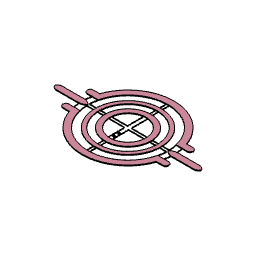
ホシノ_ヘイロー_mk1 v4 (Autodesk Fusion 360 design; units mm, degrees)
Autodesk Fusion 360 part; units mm, degrees
sketch "スケッチ1" plane through (0, 0, 0) normal (0, 0, 1) x (1, 0, 0)
  circle A0 centre (0, 0) radius 100
  circle A1 centre (0, 0) radius 82.5
  circle A2 centre (0, 0) radius 73
  circle A3 centre (0, 0) radius 57.5
  line L0 (0, 0) -> (0, 115) construction
  line L1 (0, 23) -> (-125, 23) construction
  line L2 (0, 0) -> (115, 0) construction
  line L3 (0, 38) -> (-125, 38) construction
  line L4 (-125, 23) -> (-125, 38) construction
  arc A4 (-125, 38) -> (-125, 23) centre (-125, 30.5) ccw
  line L5 (-125, 38) -> (-108.5403, 38)
  line L6 (-125, 23) -> (-112.6765, 23)
  line L7 (0, 7.5) -> (-172, 7.5) construction
  line L8 (-172, 7.5) -> (-114.7552, 7.5)
  line L9 (0, 0) -> (-190, 0) construction
  arc A5 (-172, 7.5) -> (-183.4987, 0) centre (-172, -5.0647) ccw
  line L10 (-3.5, 99.9387) -> (-3.5, 82.4257)
  line L11 (-3.5, 72.916) -> (-3.5, 57.3934)
  line L12 (3.5, 99.9387) -> (3.5, 82.4257)
  line L13 (3.5, 72.916) -> (3.5, 57.3934)
  arc A6 (-183.4987, 0) -> (-172, -7.5) centre (-172, 5.0647) ccw
  line L14 (-172, -7.5) -> (-114.7552, -7.5)
  line L15 (-125, -38) -> (-108.5403, -38)
  arc A7 (-125, -23) -> (-125, -38) centre (-125, -30.5) ccw
  line L16 (-125, -23) -> (-112.6765, -23)
  arc A8 (125, 23) -> (125, 38) centre (125, 30.5) ccw
  line L17 (125, 38) -> (108.5403, 38)
  line L18 (125, 23) -> (112.6765, 23)
  line L19 (172, 7.5) -> (114.7552, 7.5)
  arc A9 (183.4987, 0) -> (172, 7.5) centre (172, -5.0647) ccw
  arc A10 (172, -7.5) -> (183.4987, 0) centre (172, 5.0647) ccw
  line L20 (172, -7.5) -> (114.7552, -7.5)
  line L21 (125, -23) -> (112.6765, -23)
  arc A11 (125, -38) -> (125, -23) centre (125, -30.5) ccw
  line L22 (125, -38) -> (108.5403, -38)
  arc A12 (-112.6765, 23) -> (-114.7552, 7.5) centre (0, 0) ccw
  arc A13 (-114.7552, -7.5) -> (-112.6765, -23) centre (0, 0) ccw
  arc A14 (-108.5403, -38) -> (108.5403, -38) centre (0, 0) ccw
  arc A15 (112.6765, -23) -> (114.7552, -7.5) centre (0, 0) ccw
  arc A16 (114.7552, 7.5) -> (112.6765, 23) centre (0, 0) ccw
  arc A17 (108.5403, 38) -> (-108.5403, 38) centre (0, 0) ccw
  line L23 (-72.916, 3.5) -> (-57.3934, 3.5)
  line L24 (-72.916, -3.5) -> (-57.3934, -3.5)
  line L25 (-99.9387, 3.5) -> (-82.4257, 3.5)
  line L26 (-99.9387, -3.5) -> (-82.4257, -3.5)
  line L27 (-3.5, -72.916) -> (-3.5, -57.3934)
  line L28 (3.5, -72.916) -> (3.5, -57.3934)
  line L29 (-3.5, -99.9387) -> (-3.5, -82.4257)
  line L30 (3.5, -99.9387) -> (3.5, -82.4257)
  line L31 (72.916, -3.5) -> (57.3934, -3.5)
  line L32 (72.916, 3.5) -> (57.3934, 3.5)
  line L33 (99.9387, -3.5) -> (82.4257, -3.5)
  line L34 (99.9387, 3.5) -> (82.4257, 3.5)
  circle A18 centre (0, 0) radius 45
  circle A19 centre (0, -35) radius 2.6
  circle A20 centre (0, -23) radius 2.6
  line L35 (5, -44.7214) -> (5, -3.5)
  line L36 (5, 3.5) -> (5, 44.7214)
  line L37 (-5, 44.7214) -> (-5, 3.5)
  line L38 (-5, -3.5) -> (-5, -44.7214)
  line L39 (-44.8637, 3.5) -> (-5, 3.5)
  line L40 (5, 3.5) -> (44.8637, 3.5)
  line L41 (-44.8637, -3.5) -> (-5, -3.5)
  line L42 (5, -3.5) -> (44.8637, -3.5)
  arc A21 (-100, 0) -> (-114.7552, 7.5) centre (-118.3609, -17.858) ccw
  arc A22 (-114.7552, -7.5) -> (-100, 0) centre (-118.3609, 17.858) ccw
  line L43 (-112.6765, 23) -> (-97.3191, 23)
  line L44 (-112.6765, -23) -> (-97.3191, -23)
  line L45 (112.6765, 23) -> (97.3191, 23)
  arc A23 (114.7552, 7.5) -> (100, 0) centre (118.3609, -17.858) ccw
  arc A24 (100, 0) -> (114.7552, -7.5) centre (118.3609, 17.858) ccw
  line L46 (112.6765, -23) -> (97.3191, -23)
  dimension "d1" = 230
  dimension "d2" = 200
  dimension "d3" = 165
  dimension "d4" = 146
  dimension "d5" = 115
  dimension "d7" = 23
  dimension "d8" = 125
  dimension "d9" = 125
  dimension "d10" = 15
  dimension "d11" = 172
  dimension "d12" = 7
  dimension "d14" = 360
  dimension "d15" = 90
  dimension "d16" = 10
  dimension "d17" = 5.2
  dimension "d18" = 5.2
  dimension "d19" = 7.5
  constraint coincident A0.centre A1.centre
  constraint concentric A0 A1
  constraint concentric A1 A2
  constraint concentric A2 A3
  constraint coincident L0.end A12
  constraint vertical L0
  constraint coincident L0 L1.start
  constraint perpendicular L0 L1
  constraint coincident L2.end A12
  constraint horizontal L2
  constraint coincident L0 L3.start
  constraint perpendicular L0 L3
  constraint midpoint L4 A4.centre
  constraint coincident L3 L5.end
  constraint coincident L1 L6.end
  constraint coincident L0 L7.start
  constraint perpendicular L0 L7
  constraint coincident L7 L8.end
  constraint perpendicular L0 L9
  constraint tangent L7 A5
  constraint coincident L9 A5.end
  constraint coincident A0 L10.start
  constraint vertical L10
  constraint coincident A0 L12.start
  constraint symmetric L0 L10 L12
  constraint coincident A1 L10.end
  constraint coincident A2 L11.start
  constraint collinear L10 L11
  constraint coincident A1 L12.end
  constraint coincident A2 L13.start
  constraint collinear L12 L13
  constraint coincident A3 L11.end
  constraint coincident A3 L13.end
  constraint symmetric L1.end L9 A7.start
  constraint symmetric L3.end L9 L15.start
  constraint symmetric A4 L9 A7
  constraint symmetric L5.end L9 L15.end
  constraint symmetric L6.end L9 L16.end
  constraint symmetric L7.end L9 A6.end
  constraint symmetric L8.end L9 L14.end
  constraint symmetric L9 A5.end A6.start
  constraint symmetric L9 A5 A6
  constraint symmetric L0 L1.end A8.start
  constraint symmetric L0 L3.end A8.end
  constraint symmetric L0 A4 A8
  constraint symmetric L0 L5.end L17.end
  constraint symmetric L0 L6.end L18.end
  constraint symmetric L0 L7.end L19.start
  constraint symmetric L0 L8.end L19.end
  constraint symmetric L0 A5.end A9.start
  constraint symmetric L0 A5 A9
  constraint symmetric L0 A6.end A10.start
  constraint symmetric L0 A6 A10
  constraint symmetric L0 L14.end L20.end
  constraint symmetric L0 L15.start A11.start
  constraint symmetric L0 L15.end L22.end
  constraint symmetric L0 A7.start L21.start
  constraint symmetric L0 A7 A11
  constraint symmetric L0 L16.end L21.end
  constraint concentric A12 A13
  constraint concentric A13 A14
  constraint concentric A14 A15
  constraint concentric A15 A16
  constraint concentric A16 A17
  constraint concentric A0 A18
  constraint coincident A18 L37.start
  constraint coincident A18 L38.end
  constraint vertical L37
  constraint coincident A18 L35.start
  constraint coincident A18 L36.end
  constraint parallel L35 L37
  constraint coincident A18 L39.start
  constraint coincident A18 L41.start
  constraint coincident A18 L40.end
  constraint coincident A18 L42.end
  constraint coincident L36.start L39
  constraint collinear L35 L36
  constraint coincident L35.end L41
  constraint collinear L37 L38
  constraint collinear L39 L40
  constraint collinear L41 L42
  constraint coincident A0 A21.start
  constraint coincident L9 A21.start
  constraint symmetric L9 A21.start A22.end
  constraint symmetric L9 A21 A22
  constraint coincident A0 L43.end
  constraint coincident L1 L43.end
  constraint coincident A0 L44.end
  constraint parallel L16 L44
  constraint symmetric L0 A21.start A23.end
  constraint symmetric L0 A21 A23
  constraint symmetric L0 A22 A24
  constraint symmetric L0 L43.end L45.end
  constraint symmetric L0 L44.end L46.end
  measures "d1" diameter of A12
  measures "d2" diameter of A0
  measures "d3" diameter of A1
  measures "d4" diameter of A2
  measures "d5" diameter of A3
  measures "d7" distance of L1 L2
  measures "d8" distance of L1.start L1.end
  measures "d9" distance of L3.start L3.end
  measures "d10" distance of L1 L3
  measures "d11" distance of L7.start L7.end
  measures "d12" distance of L10 L12
  measures "d15" diameter of A18
  measures "d16" distance of L35 L37
  measures "d17" diameter of A19
  measures "d18" diameter of A20
  measures "d19" distance of L7 L9
extrude "押し出し1" add sketch "スケッチ1" along normal blind 2 contours L19 A9 A10 L20 A23 A24 | A0 A4 L5 L6 A8 L17 L18 A17 L43 L45 | A1 | A0 L15 A7 L16 L21 A11 L22 A14 L44 L46 | L8 A5 A6 L14 A21 A22 | A3 makes body 1 at (-133.8368, -2.5, 0) makes body 2 at (-110.2865, 28, 2) makes body 3 at (110.2865, -28, 2) makes body 4 at (-49.9173, 18.3869, 0) makes body 5 at (-77.5326, -15.8311, 0) makes body 6 at (133.8368, 2.5, 0)
extrude "押し出し2" add sketch "スケッチ1" along normal blind 2 separate body contours A0 A1 L33 L34 | A0 A15 A24 L46 | A0 A16 L45 A23 | A0 A1 L10 L12 | A0 A1 L29 L30 | A0 A12 A21 L43 | A0 A1 L25 L26 | A0 A13 A22 L44 | A2 A3 L31 L32 | A2 A3 L11 L13 | A2 A3 L27 L28 | A2 A3 L23 L24 | A18 L35 L36 L37 L38 L39 L40 L41 L42 makes body 7 at (2.7223, -88.2854, 0) makes body 8 at (0.5566, 17.323, 2) makes body 9 at (-62.5992, 2.7224, 0) makes body 10 at (-2.7224, -62.5992, 0) makes body 11 at (62.5992, -2.7224, 0) makes body 12 at (2.7224, 62.5992, 0) makes body 13 at (-102.8715, -20.854, 0) makes body 14 at (2.7223, 88.2854, 0) makes body 15 at (102.8715, 20.854, 0)
